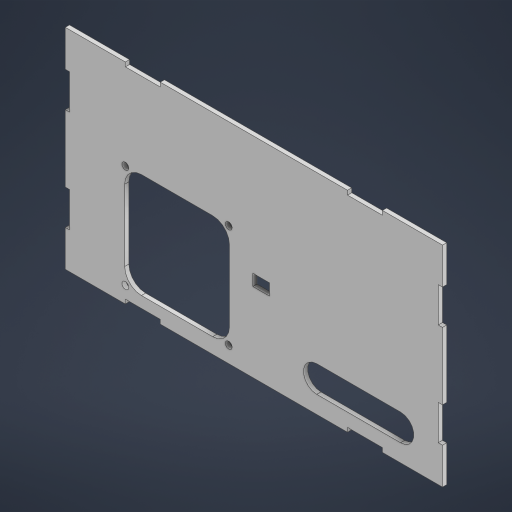
# Autodesk Inventor part: side_part
Saved by Autodesk Inventor 2023 (Build 270158000, 158)
## iProperties
Created: 2022-11-27
Part Number: side_part
Material: Generic
Document SubType Name: Modeling
Designer: washington
Density: 1 g/cm^3
Appearance: Default
Author: washington
Autodesk Inventor part; units mm, degrees
ref_plane "YZ Plane" through (0, 0, 0) normal (1, 0, 0) x (0, 1, 0)
ref_plane "XZ Plane" through (0, 0, 0) normal (0, 1, 0) x (-1, 0, 0)
ref_plane "XY Plane" through (0, 0, 0) normal (0, 0, 1) x (1, 0, 0)
sketch "Sketch1" plane through (0, 0, 0) normal (0, 0, 1) x (1, 0, 0)
  line L0 (135, 75) -> (-135, 75)
  line L1 (-135, -75) -> (135, 75) construction
  line L2 (135, -75) -> (-135, 75) construction
  line L3 (-80.5, 11) -> (-29.5, 11)
  line L4 (-17.5, -1) -> (-17.5, -52)
  line L5 (-29.5, -64) -> (-80.5, -64)
  line L6 (-92.5, -52) -> (-92.5, -1)
  line L7 (-92.5, 11) -> (-17.5, -64) construction
  line L8 (-17.5, 11) -> (-92.5, -64) construction
  line L9 (45, -53) -> (105, -53) construction
  line L10 (45, -62.5) -> (105, -62.5)
  line L11 (105, -43.5) -> (45, -43.5)
  arc A0 (45, -43.5) -> (45, -62.5) centre (45, -53) ccw
  arc A1 (105, -62.5) -> (105, -43.5) centre (105, -53) ccw
  line L12 (135, -49) -> (132, -49)
  line L13 (132, -49) -> (132, -24)
  line L14 (132, -24) -> (135, -24)
  line L15 (0, 0) -> (156, 0) construction
  line L16 (135, 49) -> (132, 49)
  line L17 (132, 49) -> (132, 24)
  line L18 (132, 24) -> (135, 24)
  line L19 (135, 49) -> (135, 75)
  line L20 (135, -75) -> (135, -49)
  line L21 (135, -24) -> (135, 24)
  line L22 (-135, 49) -> (-132, 49)
  line L23 (-132, 49) -> (-132, 24)
  line L24 (-132, 24) -> (-135, 24)
  line L25 (0, 0) -> (-98, 0)
  line L26 (-135, 75) -> (-135, 49)
  line L27 (-135, -49) -> (-132, -49)
  line L28 (-132, -49) -> (-132, -24)
  line L29 (-132, -24) -> (-135, -24)
  line L30 (-135, 24) -> (-135, -24)
  line L31 (-135, -49) -> (-135, -75)
  line L32 (-92, -75) -> (-92, -72)
  line L33 (-92, -72) -> (-67, -72)
  line L34 (-67, -72) -> (-67, -75)
  line L35 (-135, -75) -> (-92, -75)
  line L36 (0, 0) -> (0, 97)
  line L37 (92, -75) -> (92, -72)
  line L38 (92, -72) -> (67, -72)
  line L39 (67, -72) -> (67, -75)
  line L40 (-67, -75) -> (67, -75)
  line L41 (92, -75) -> (135, -75)
  line L42 (-95, 13.5) -> (-15, 13.5) construction
  line L43 (-15, 13.5) -> (-15, -66.5) construction
  line L44 (-15, -66.5) -> (-95, -66.5) construction
  line L45 (-95, -66.5) -> (-95, 13.5) construction
  line L46 (-95, 13.5) -> (-15, -66.5) construction
  line L47 (-15, 13.5) -> (-95, -66.5) construction
  circle A2 centre (-92, 10.5) radius 2.5
  arc A3 (-80.5, 11) -> (-92.5, -1) centre (-80.5, -1) ccw
  arc A4 (-17.5, -1) -> (-29.5, 11) centre (-29.5, -1) ccw
  arc A5 (-29.5, -64) -> (-17.5, -52) centre (-29.5, -52) ccw
  arc A6 (-92.5, -52) -> (-80.5, -64) centre (-80.5, -52) ccw
  circle A7 centre (-18, 10.5) radius 2.5
  circle A8 centre (-92, -63.5) radius 2.5
  circle A9 centre (-18, -63.5) radius 2.5
  line L48 (-0.75, -10.3) -> (11.15, -10.3)
  line L49 (11.15, -10.3) -> (11.15, -18.5)
  line L50 (11.15, -18.5) -> (-0.75, -18.5)
  line L51 (-0.75, -18.5) -> (-0.75, -10.3)
  line L52 (-0.75, -10.3) -> (11.15, -18.5) construction
  line L53 (11.15, -10.3) -> (-0.75, -18.5) construction
  line L54 (0, 0) -> (187, 0)
  line L55 (-92, 75) -> (-92, 72)
  line L56 (-92, 72) -> (-67, 72)
  line L57 (-67, 72) -> (-67, 75)
  line L58 (92, 75) -> (92, 72)
  line L59 (92, 72) -> (67, 72)
  line L60 (67, 72) -> (67, 75)
  point P0 (-55, -26.5)
  point P1 (25, -75)
  point P2 (75, -53)
  point P3 (5.2, -14.4)
  dimension "d0" = 150
  dimension "d1" = 270
  dimension "d2" = 75
  dimension "d3" = 75
  dimension "d4" = 55
  dimension "d5" = 11
  dimension "d6" = 22
  dimension "d7" = 210
  dimension "d8" = 9.5
  dimension "d9" = 20
  dimension "d12" = 26
  dimension "d13" = 3
  dimension "d14" = 25
  dimension "d15" = 0
  dimension "d16" = 21
  dimension "d17" = 3
  dimension "d18" = 25
  dimension "d19" = 26
  dimension "d20" = 270
  dimension "d21" = 233
  dimension "d22" = 25
  dimension "d23" = 3
  dimension "d24" = 43
  dimension "d25" = 30
  dimension "d26" = 124
  dimension "d27" = 48
  dimension "d28" = 80
  dimension "d29" = 5
  dimension "d30" = 3
  dimension "d31" = 12
  dimension "d32" = 12
  dimension "d33" = 12
  dimension "d34" = 5
  dimension "d35" = 3
  dimension "d36" = 3
  dimension "d37" = 5
  dimension "d38" = 3
  dimension "d39" = 3
  dimension "d40" = 5
  dimension "d41" = 3
  dimension "d42" = 11.9
  dimension "d43" = 8.2
  dimension "d44" = 14.4
  dimension "d45" = 5.2
  constraints: 124 end point, 23 perpendicular, 20 symmetric about line, 19 parallel, 12 horizontal, 12 point on circle, 12 point on line, 12 tangent, 10 centre point, 9 midpoint, 1 equal radius, 1 vertical
  measures "d0" distance of L2.start L0.start
  measures "d1" distance of L1.start L2.start
  measures "d2" distance of L8.start L7.end
  measures "d3" distance of L7.end L8.end
  measures "d4" horizontal distance of point (-55, -26.5) L15.start
  measures "d5" distance from line of L5 point (25, -75)
  measures "d6" vertical distance of L9.end L2.start
  measures "d7" horizontal distance of L1.start point (75, -53)
  measures "d8" radius of A1
  measures "d9" horizontal distance of point (25, -75) L9.start
  measures "d12" distance from line of L12 L2.start
  measures "d13" distance of L13.end L14.end
  measures "d14" distance of L12.end L13.end
  measures "d15" distance between parallel lines of L21 L19
  measures "d16" distance from line of L15.end L19
  measures "d17" distance of L22.start L22.end
  measures "d18" distance between parallel lines of L22 L24
  measures "d19" distance between parallel lines of L0 L22
  measures "d20" distance between parallel lines of L30 L19
  measures "d21" distance from line of L25.end L20
  measures "d22" distance of L32.end L33.end
  measures "d23" distance of L32.start L32.end
  measures "d24" horizontal distance of L1.start L32.end
  measures "d25" distance from line of L11.start L19
  measures "d26" distance between parallel lines of L16 L40
  measures "d27" distance from line of L36.end L16
  measures "d28" distance of L42.end L43.end
  measures "d29" diameter of A2
  measures "d30" distance from line of A2.centre L45
  measures "d31" radius of A3
  measures "d32" radius of A4
  measures "d33" radius of A5
  measures "d34" diameter of A7
  measures "d35" distance from line of L42 A7.centre
  measures "d36" distance from line of L43 A7.centre
  measures "d37" diameter of A8
  measures "d38" horizontal distance of A8.centre L44.end
  measures "d39" distance from line of A8.centre L44
  measures "d40" diameter of A9
  measures "d41" distance from line of A9.centre L44
  measures "d42" distance of L49.end L50.end
  measures "d43" distance of L48.end L49.end
  measures "d44" vertical distance of point (5.2, -14.4) L15.start
  measures "d45" horizontal distance of L15.start point (5.2, -14.4)
extrude "Extrusion1" add sketch "Sketch1" along normal blind 3 contours L19 L16 L17 L18 L21 L54 L36 L0 L60 L59 L58 | L36 L54 L21 L14 L13 L12 L20 L41 L37 L38 L39 L40 L34 L33 L32 L35 L31 L27 L28 L29 L30 L24 L23 L22 L26 L0 L55 L56 L57
body "Solid1"
